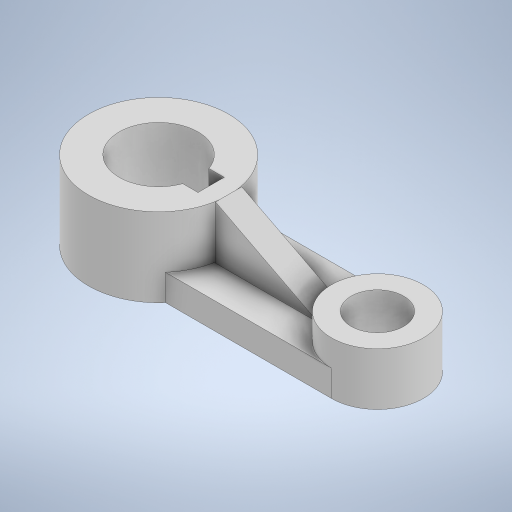
# Autodesk Inventor part: 6 -  Part 4
Saved by Autodesk Inventor 2024 (Build 280153000, 153)
## iProperties
Created: 2024-04-21
Part Number: 6 -  Part 4
Material: Generic
Document SubType Name: Modeling
Designer: Ricsi
Density: 1 g/cm^3
Appearance: Default
Author: Ricsi
Autodesk Inventor part; units mm, degrees
ref_plane "YZ Plane" through (0, 0, 0) normal (1, 0, 0) x (0, 1, 0)
ref_plane "XZ Plane" through (0, 0, 0) normal (0, 1, 0) x (-1, 0, 0)
ref_plane "XY Plane" through (0, 0, 0) normal (0, 0, 1) x (1, 0, 0)
sketch "Sketch1" plane through (0, 0, 0) normal (0, 1, 0) x (-1, 0, 0)
  arc A0 (-16.9706, -6) -> (-16.9706, 6) centre (0, 0) ccw
  circle A1 centre (0, 0) radius 32
  line L0 (-24, 0) -> (-24, 6)
  line L1 (-24, 0) -> (-24, -6)
  line L2 (-24, 6) -> (-16.9706, 6)
  line L3 (-24, -6) -> (-16.9706, -6)
  circle A2 centre (-100, 0) radius 12
  circle A3 centre (-100, 0) radius 21
  dimension "d0" = 36
  dimension "d1" = 64
  dimension "d3" = 6
  dimension "d4" = 6
  dimension "d6" = 24
  dimension "d7" = 42
  constraints: 8 end point, 4 centre point, 3 coincident, 2 horizontal, 2 point on circle, 2 vertical
  measures "d0" diameter of A0
  measures "d1" diameter of A1
  measures "d3" distance of L0.start L0.end
  measures "d4" distance of L0.start L1.end
  measures "d6" diameter of A2
  measures "d7" diameter of A3
extrude "Extrusion1" add sketch "Sketch1" along normal blind 36
sketch "Sketch2" plane through (100, 36, 0) normal (0, 1, 0) x (1, 0, 0)
  circle A0 centre (0, 0) radius 12 projected
  circle A1 centre (0, 0) radius 21
  point P0 (-100, 0)
  dimension "d10" = 42
  constraints: 1 centre point, 1 coincident
  measures "d10" diameter of A1
extrude "Extrusion2" cut sketch "Sketch2" against normal blind 12
sketch "Sketch3" plane through (0, 0, 0) normal (0, 1, 0) x (-1, 0, 0)
  circle A0 centre (-100, 0) radius 21 projected
  line L0 (-100, -21) -> (-24.1454, -21)
  circle A1 centre (0, 0) radius 32 projected
  line L1 (-100, 21) -> (-24.1454, 21)
  arc A2 (-100, -21) -> (-100, 21) centre (-100, 0) ccw
  circle A3 centre (0, 0) radius 30.971
  circle A4 centre (0, 0) radius 32
  circle A5 centre (-100, 0) radius 21
  dimension "d14" = 64
  constraints: 6 point on circle, 4 centre point, 4 coincident, 4 end point, 1 horizontal
  measures "d14" diameter of A4
extrude "Extrusion3" add sketch "Sketch3" along normal blind 12 contours A0 L1 A1 L0
sketch "Sketch4" plane through (0, 12, 0) normal (0, 1, 0) x (1, 0, 0)
  arc A0 (24.1454, -21) -> (24.1454, 21) centre (0, 0) ccw projected
  line L0 (32, 0) -> (32, -6)
  line L1 (32, 0) -> (32, 6)
  arc A1 (100, 21) -> (100, -21) centre (100, 0) ccw projected
  line L2 (79, 0) -> (79, 6)
  line L3 (79, 0) -> (79, -6)
  line L4 (32, 6) -> (79, 6)
  line L5 (32, -6) -> (79, -6)
  dimension "d17" = 6
  dimension "d18" = 6
  dimension "d19" = 6
  dimension "d20" = 6
  constraints: 12 end point, 4 vertical, 2 point on circle, 2 tangent
  measures "d17" distance of L0.start L0.end
  measures "d18" distance of L0.start L1.end
  measures "d19" distance of L2.start L2.end
  measures "d20" distance of L2.start L3.end
extrude "Extrusion4" add sketch "Sketch4" along normal blind 24.25
sketch "Sketch5" plane through (79, 12, -6) normal (0, 0, -1) x (-1, 0, 0)
  line L0 (0, 0) -> (0, 24.25) projected
  line L1 (0, 0) -> (47, 24.25)
  line L2 (47, 24.25) -> (0, 24.25)
  line L3 (0, 0) -> (-21, 0) projected
  line L4 (0, 24.25) -> (0, 0)
  point P0 (79, -12)
  constraints: 6 end point, 1 horizontal, 1 perpendicular
extrude "Extrusion5" cut sketch "Sketch5" against normal blind 24.25
body "Solid1"
